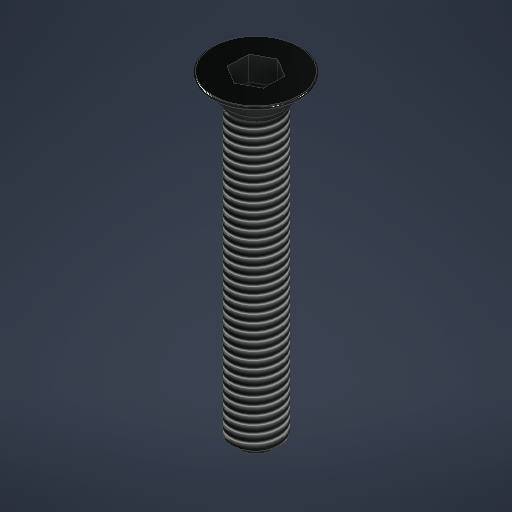
# Autodesk Inventor part: Screw M3 8mm flat head
Saved by Autodesk Inventor 2026.2 (Build 302298000, 298)
## iProperties
Created: 2026-03-09
Part Number: Screw M3 8mm flat head
Material: Ogólny
Document SubType Name: Modeling
Designer: idzim
Density: 1 g/cm^3
Appearance: Domyślna
Author: idzim
Autodesk Inventor part; units mm, degrees
ref_plane "YZ Plane" through (0, 0, 0) normal (1, 0, 0) x (0, 1, 0)
ref_plane "XZ Plane" through (0, 0, 0) normal (0, 1, 0) x (-1, 0, 0)
ref_plane "XY Plane" through (0, 0, 0) normal (0, 0, 1) x (1, 0, 0)
sketch "Szkic2" plane through (0, 0, 0) normal (1, 0, 0) x (0, 1, 0)
  line L0 (0, -2.9) -> (0, 2.9)
  line L1 (-1.5, -1.5) -> (-1.5, 1.5)
  line L2 (-1.5, -1.5) -> (0, -2.9)
  line L3 (-1.5, 1.5) -> (0, 2.9)
  line L4 (0, 0) -> (-20, 0)
  line L5 (-20, 0) -> (-20, -1.5)
  line L6 (-20, -1.5) -> (-1.5, -1.5)
  dimension "d0" = 5.8
  dimension "d2" = 3
  dimension "d3" = 1.5
  dimension "d4" = 20
  dimension "d5" = 1.5
  constraints: 14 end point, 2 perpendicular, 2 vertical, 1 horizontal, 1 midpoint
  measures "d0" distance of L0.start L0.end
  measures "d2" distance of L1.start L1.end
  measures "d3" distance between parallel lines of L0 L1
  measures "d4" distance of L4.start L4.end
  measures "d5" distance of L4.end L5.end
revolve "Obrót1" add sketch "Szkic2" angle 360 about axis through (0, 0, 0) along (0, -1, 0) contours L2 L1 L4 L0 | L6 L5 L4 L1
sketch "Szkic3" plane through (0, 0, 0) normal (0, 1, 0) x (1, 0, 0)
  line L0 (-1.1673, -0.633) -> (-1.1318, 0.6945)
  line L1 (-1.1318, 0.6945) -> (0.0355, 1.3274)
  line L2 (0.0355, 1.3274) -> (1.1673, 0.633)
  line L3 (1.1673, 0.633) -> (1.1318, -0.6945)
  line L4 (1.1318, -0.6945) -> (-0.0355, -1.3274)
  line L5 (-0.0355, -1.3274) -> (-1.1673, -0.633)
  point P0 (0, 0)
  point P1 (0, 0)
  dimension "d7" = 2.3
  constraints: 12 end point, 1 coincident, 13 other
  measures "d7" distance between parallel lines of L3 L0
extrude "Wyciągnięcie proste1" cut sketch "Szkic3" against normal blind 2
fillet "Zaokrąglenie1" radius 0.5 6 edges at (-1.1496, -2, -0.0308) (-0.6014, -2, 0.9802) (-0.5482, -2, -1.011) (0.6014, -2, -0.9802) (0.5482, -2, 1.011) (1.1496, -2, 0.0308)
fillet "Zaokrąglenie2" radius 0.5 1 edges at (0, -1.5, 1.5)
fillet "Zaokrąglenie3" radius 0.1 1 edges at (0, 0, 2.9)
thread "Gwint1" size "M3x0.5" class "6g" standard "ANSI Metric M Profile" full length
chamfer "Faza1" distance 0.5 angle 45 1 edges at (0, -20, 1.5)
